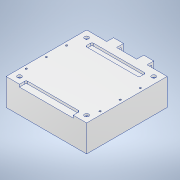
# Autodesk Inventor part: Base - V1
Saved by Autodesk Inventor 2022 (Build 260153000, 153)
## iProperties
Created: 2022-06-13
Part Number: Base - V1
Material: Aluminum 6061
Document SubType Name: Modeling
Designer: Caleb
Density: 2.7 g/cm^3
Appearance: Aluminum - Flat
Mass: 397.038 g
Surface Area: 211.278 cm^2
Volume: 147.051 cm^3
Author: Caleb
Autodesk Inventor part; units mm, degrees
ref_plane "YZ Plane" through (0, 0, 0) normal (1, 0, 0) x (0, 1, 0)
ref_plane "XZ Plane" through (0, 0, 0) normal (0, 1, 0) x (-1, 0, 0)
ref_plane "XY Plane" through (0, 0, 0) normal (0, 0, 1) x (1, 0, 0)
sketch "Sketch1" plane through (0, 0, 0) normal (0, 1, 0) x (-1, 0, 0)
  line L0 (-38.1, -41.275) -> (38.1, -41.275)
  line L1 (38.1, -41.275) -> (38.1, 41.275)
  line L2 (38.1, 41.275) -> (-38.1, 41.275)
  line L3 (-38.1, 41.275) -> (-38.1, -41.275)
  line L4 (-38.1, -41.275) -> (38.1, 41.275) construction
  line L5 (38.1, -41.275) -> (-38.1, 41.275) construction
  point P0 (0, 0)
  dimension "d0" = 76.2
  dimension "d1" = 82.55
  constraints: 12 end point, 2 midpoint, 2 parallel, 1 horizontal, 1 perpendicular
  measures "d0" distance of L2.end L1.end
  measures "d1" distance of L1.end L0.end
extrude "Extrusion1" add sketch "Sketch1" along normal blind 25.4
sketch "Sketch2" plane through (0, 25.4, 0) normal (0, 1, 0) x (1, 0, 0)
  line L0 (9.525, 34.671) -> (9.525, 41.275)
  line L1 (9.525, 41.275) -> (-9.525, 41.275)
  line L2 (-9.525, 41.275) -> (-9.525, 34.671)
  line L3 (-9.525, 34.671) -> (9.525, 34.671)
  line L4 (9.525, 34.671) -> (-9.525, 41.275) construction
  line L5 (9.525, 41.275) -> (-9.525, 34.671) construction
  line L6 (-38.1, 41.275) -> (-38.1, -41.275) projected
  line L7 (-38.1, 41.275) -> (-19.05, 41.275)
  line L8 (-19.05, 41.275) -> (-19.05, 34.925)
  line L9 (-19.05, 34.925) -> (-38.1, 34.925)
  line L10 (-38.1, 34.925) -> (-38.1, 41.275)
  line L11 (38.1, -41.275) -> (38.1, 41.275) projected
  line L12 (38.1, 41.275) -> (19.05, 41.275)
  line L13 (19.05, 41.275) -> (19.05, 34.925)
  line L14 (19.05, 34.925) -> (38.1, 34.925)
  line L15 (38.1, 34.925) -> (38.1, 41.275)
  line L16 (38.1, 41.275) -> (-38.1, 41.275) projected
  point P0 (0, 0)
  point P1 (0, 37.973)
  dimension "d6" = 9.525
  dimension "d7" = 9.525
  dimension "d8" = 6.35
  dimension "d9" = 19.05
  dimension "d58" = 6.604
  constraints: 28 end point, 6 parallel, 3 perpendicular, 2 horizontal, 2 midpoint, 2 point on line, 1 collinear
  measures "d6" distance between parallel lines of L8 L2
  measures "d7" distance between parallel lines of L0 L13
  measures "d8" distance of L9.end L6.start
  measures "d9" distance of L2.end L0.start
  measures "d58" distance of L1.end L2.end
extrude "Extrusion2" cut sketch "Sketch2" against normal through all
sketch "Sketch3" plane through (19.05, 25.4, -34.925) normal (1, 0, 0) x (0, 0, -1)
  line L0 (-0.254, 0) -> (-0.254, -25.4) projected
  line L1 (6.35, -25.4) -> (-0.254, -25.4)
  line L2 (-0.254, -25.4) -> (-0.254, -12.7)
  line L3 (-0.254, -12.7) -> (6.35, -12.7)
  line L4 (6.35, -12.7) -> (6.35, -25.4)
  point P0 (-34.925, -25.4)
  constraints: 8 end point, 2 parallel, 1 horizontal, 1 midpoint, 1 perpendicular
extrude "Extrusion3" cut sketch "Sketch3" against normal through all
sketch "Sketch4" plane through (19.05, 25.4, -34.925) normal (1, 0, 0) x (0, 0, -1)
  line L0 (0, 0) -> (6.35, 0) projected
  line L1 (6.35, 0) -> (6.35, -12.7) projected
  point P0 (-34.925, -25.4)
  point P1 (3.175, -3.175)
  dimension "d14" = 3.175
  dimension "d15" = 3.175
  measures "d14" distance from line of L0 point (3.175, -3.175)
  measures "d15" distance from line of point (3.175, -3.175) L1
hole "Hole1" at (19.05, 22.225, -38.1) direction (-1, 0, 0) diameter 2.54 end through all
sketch "Sketch6" plane through (0, 25.4, 0) normal (0, 1, 0) x (1, 0, 0)
  line L0 (-23.8125, 27.305) -> (23.8125, 27.305)
  line L1 (25.4, 25.7175) -> (25.4, 22.5425)
  line L2 (23.8125, 20.955) -> (-23.8125, 20.955)
  line L3 (-25.4, 22.5425) -> (-25.4, 25.7175)
  line L4 (-38.1, 34.925) -> (-38.1, -41.275) projected
  line L5 (-38.1, -41.275) -> (38.1, -41.275) projected
  line L6 (-25.4, -41.275) -> (25.4, -41.275)
  line L7 (25.4, -41.275) -> (25.4, -36.5125)
  line L8 (23.8125, -34.925) -> (-23.8125, -34.925)
  line L9 (-25.4, -36.5125) -> (-25.4, -41.275)
  arc A0 (-23.8125, -34.925) -> (-25.4, -36.5125) centre (-23.8125, -36.5125) ccw
  arc A1 (25.4, -36.5125) -> (23.8125, -34.925) centre (23.8125, -36.5125) ccw
  arc A2 (23.8125, 20.955) -> (25.4, 22.5425) centre (23.8125, 22.5425) ccw
  arc A3 (25.4, 25.7175) -> (23.8125, 27.305) centre (23.8125, 25.7175) ccw
  arc A4 (-23.8125, 27.305) -> (-25.4, 25.7175) centre (-23.8125, 25.7175) ccw
  arc A5 (-25.4, 22.5425) -> (-23.8125, 20.955) centre (-23.8125, 22.5425) ccw
  line L10 (-19.05, 34.925) -> (-38.1, 34.925) projected
  point P0 (0, 0)
  point P1 (-25.4, 27.305)
  point P2 (-38.1, 31.75)
  point P3 (38.1, 31.75)
  point P4 (25.4, 20.955)
  point P5 (25.4, 27.305)
  point P6 (-25.4, 20.955)
  point P7 (25.4, -34.925)
  point P8 (-25.4, -34.925)
  point P9 (25.4, -41.275)
  dimension "d25" = 50.8
  dimension "d26" = 6.35
  dimension "d28" = 12.7
  dimension "d29" = 50.8
  dimension "d30" = 6.35
  dimension "d31" = 12.7
  dimension "d46" = 1.5875
  dimension "d60" = 7.62
  constraints: 16 end point, 13 point on line, 12 point on circle, 12 tangent, 6 centre point, 5 equal radius, 4 parallel, 2 horizontal, 2 perpendicular
  measures "d25" distance of point (25.4, 20.955) point (-25.4, 20.955)
  measures "d26" distance of point (25.4, 27.305) point (25.4, 20.955)
  measures "d28" distance between parallel lines of L4 L3
  measures "d29" distance of point (-25.4, -34.925) point (25.4, -34.925)
  measures "d30" distance of point (25.4, -34.925) L6.end
  measures "d31" distance between parallel lines of L4 L9
  measures "d46" radius of A0
  measures "d60" distance between parallel lines of L10 L0
extrude "Extrusion5" cut sketch "Sketch6" against normal blind 2.3813
sketch "Sketch7" plane through (0, 25.4, 0) normal (0, 1, 0) x (1, 0, 0)
  line L0 (38.1, -41.275) -> (38.1, 34.925) projected
  line L1 (0, -14.8069) -> (0, 17.784) construction
  line L2 (25.4, -41.275) -> (38.1, -41.275) projected
  point P0 (0, 0)
  point P1 (34.925, -6.35)
  point P2 (34.925, -25.4)
  point P3 (34.925, 12.7)
  point P4 (38.1, 31.75)
  point P5 (-34.925, -6.35)
  point P6 (-34.925, -25.4)
  point P7 (-34.925, 12.7)
  dimension "d34" = 19.05
  dimension "d35" = 19.05
  dimension "d36" = 3.175
  dimension "d44" = 34.925
  constraints: 3 symmetric about line, 2 end point, 2 vertical alignment, 1 vertical
  measures "d34" distance of point (34.925, -25.4) point (34.925, -6.35)
  measures "d35" distance of point (34.925, 12.7) point (34.925, -6.35)
  measures "d36" distance from line of L0 point (34.925, -6.35)
  measures "d44" distance from line of L2 point (34.925, -6.35)
hole "Hole2" at (34.925, 25.4, 6.35) at (34.925, 25.4, 25.4) at (34.925, 25.4, -12.7) at (-34.925, 25.4, -12.7) at (-34.925, 25.4, 25.4) at (-34.925, 25.4, 6.35) direction (0, -1, 0) diameter 1.6942 end through all thread size "2-56 UNC" class "2B" standard "ANSI Unified Screw Threads"
sketch "Sketch8" plane through (0, 25.4, 0) normal (0, 1, 0) x (1, 0, 0)
  line L0 (-38.1, 34.925) -> (-38.1, -41.275) projected
  line L1 (-38.1, -41.275) -> (-25.4, -41.275) projected
  line L2 (38.1, -41.275) -> (38.1, 34.925) projected
  line L3 (38.1, 34.925) -> (19.05, 34.925) projected
  point P0 (0, 0)
  point P1 (-31.75, -34.925)
  point P2 (-31.75, 28.575)
  point P3 (31.75, 28.575)
  point P4 (31.75, -34.925)
  dimension "d47" = 6.35
  dimension "d48" = 6.35
  dimension "d50" = 6.35
  dimension "d61" = 6.35
  constraints: 2 horizontal alignment, 2 vertical alignment
  measures "d47" distance from line of L0 point (-31.75, -34.925)
  measures "d48" distance from line of L1 point (-31.75, -34.925)
  measures "d50" distance from line of L2 point (31.75, 28.575)
  measures "d61" distance from line of L3 point (31.75, 28.575)
hole "Hole3" at (-31.75, 25.4, 34.925) at (-31.75, 25.4, -28.575) at (31.75, 25.4, -28.575) at (31.75, 25.4, 34.925) direction (0, -1, 0) diameter 2.0574 end through all counterbore diameter 3.9624 counterbore depth 1.8542 clearance for "Socket Head Cap Screw" size "#1" standard "Ansi Unified Screw Threads"
equation "\"d7\" = d6"
equation "\"d15\" = d14"
equation "\"d31\" = d28"
equation "\"d47\" = d48"
equation "\"d50\" = d48"
equation "\"d61\" = d48"
body "Solid1"
